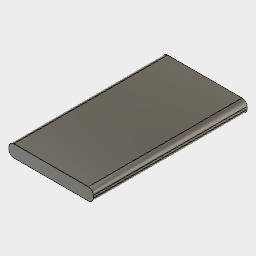
258 1200mAh lipo (Autodesk Fusion 360 design; units mm, degrees)
Autodesk Fusion 360 part; units mm, degrees
sketch "Sketch1" plane through (0, 0, 0) normal (0, 0, 1) x (1, 0, 0)
box "BoxPrimitive1" add length 62 width 34 height 5 placed x (0, 1, 0) y (-1, 0, 0) z (0, 0, 1) at (34, 0, 0)
fillet "Fillet1" radius 2 4 edges at (34, 31, 5) (34, 31, 0) (0, 31, 5) (0, 31, 0)
